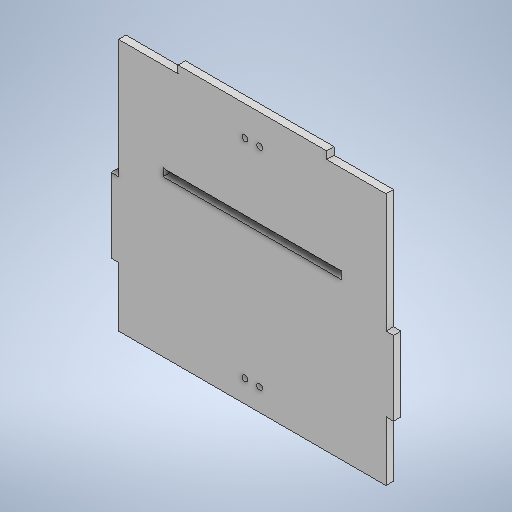
# Autodesk Inventor part: back
Saved by Autodesk Inventor 2025.3 (Build 293356030, 356C)
## iProperties
Created: 2026-06-26
Part Number: back
Material: Generic
Document SubType Name: Modeling
Designer: user
Density: 1 g/cm^3
Appearance: Default
Author: user
Autodesk Inventor part; units mm, degrees
ref_plane "YZ Plane" through (0, 0, 0) normal (1, 0, 0) x (0, 1, 0)
ref_plane "XZ Plane" through (0, 0, 0) normal (0, 1, 0) x (-1, 0, 0)
ref_plane "XY Plane" through (0, 0, 0) normal (0, 0, 1) x (1, 0, 0)
sketch "Sketch1" plane through (0, 0, 0) normal (0, 0, 1) x (1, 0, 0)
  line L0 (0, 0) -> (180, 0)
  line L1 (180, 0) -> (180, 170)
  line L2 (180, 170) -> (0, 170)
  line L3 (0, 170) -> (0, 0)
  line L4 (0, 40) -> (-5, 40)
  line L5 (-5, 40) -> (-5, 90)
  line L6 (-5, 90) -> (0, 90)
  line L7 (0, 90) -> (0, 40)
  line L8 (90, 0) -> (90, 170) construction
  line L9 (180, 40) -> (185, 40)
  line L10 (185, 40) -> (185, 90)
  line L11 (185, 90) -> (180, 90)
  line L12 (180, 90) -> (180, 40)
  line L13 (30, 105) -> (150, 105)
  line L14 (150, 105) -> (150, 110)
  line L15 (150, 110) -> (30, 110)
  line L16 (30, 110) -> (30, 105)
  line L17 (0, 65) -> (180, 65) construction
  line L18 (40, 170) -> (140, 170)
  line L19 (140, 170) -> (140, 175)
  line L20 (140, 175) -> (40, 175)
  line L21 (40, 175) -> (40, 170)
  point P0 (180, 40)
  point P1 (180, 90)
  point P2 (0, 90)
  point P3 (40, 0)
  point P4 (30, 107.5)
  dimension "d0" = 180
  dimension "d1" = 170
  dimension "d2" = 5
  dimension "d3" = 50
  dimension "d6" = 120
  dimension "d7" = 5
  dimension "d13" = 60
  dimension "d14" = 60
  dimension "d30" = 100
  dimension "d31" = 5
  dimension "d32" = 40
  constraints: 44 end point, 8 parallel, 5 midpoint, 4 horizontal, 4 perpendicular, 4 symmetric about line, 3 point on line
  measures "d0" distance of L2.end L1.end
  measures "d1" distance of L1.end L0.end
  measures "d2" distance of L5.end L6.end
  measures "d3" distance of L4.end L5.end
  measures "d6" distance of L15.end L14.end
  measures "d7" distance of L14.end L13.end
  measures "d13" distance between parallel lines of L2 L15
  measures "d14" distance from line of point (30, 107.5) L8
  measures "d30" distance of L20.end L19.end
  measures "d31" distance of L19.end L18.end
  measures "d32" distance between parallel lines of L1 L19
extrude "Extrusion1" add sketch "Sketch1" along normal blind 5
sketch "Sketch2" plane through (0, 0, 5) normal (0, 0, 1) x (1, 0, 0)
  line L0 (180, 170) -> (0, 170) projected
  line L1 (0, 0) -> (180, 0) projected
  line L2 (0, 170) -> (0, 90) projected
  line L3 (0, 40) -> (0, 0) projected
  point P0 (85, 15)
  point P1 (95, 15)
  dimension "d24" = 15
  dimension "d25" = 15
  dimension "d26" = 10
  dimension "d29" = 85
  measures "d24" distance from line of L1 point (85, 15)
  measures "d25" distance from line of L1 point (95, 15)
  measures "d26" distance of point (95, 15) point (85, 15)
  measures "d29" distance from line of L3 point (85, 15)
hole "Hole1" at (85, 15, 5) at (95, 15, 5) direction (0, 0, -1) diameter 4 end through all
sketch "Sketch3" plane through (0, 0, 5) normal (0, 0, 1) x (1, 0, 0)
  line L0 (140, 175) -> (40, 175) projected
  line L1 (40, 175) -> (40, 170) projected
  point P0 (0, 0)
  point P1 (85, 155)
  point P2 (95, 155)
  dimension "d40" = 20
  dimension "d41" = 20
  dimension "d42" = 10
  dimension "d43" = 45
  measures "d40" distance from line of point (85, 155) L0
  measures "d41" distance from line of L0 point (95, 155)
  measures "d42" distance of point (95, 155) point (85, 155)
  measures "d43" distance from line of point (85, 155) L1
hole "Hole2" at (85, 155, 5) at (95, 155, 5) direction (0, 0, -1) diameter 4 end through all
body "Solid1"
